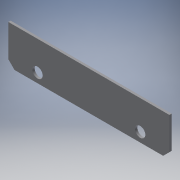
# Autodesk Inventor part: MecanumDriveTrainPlate17-18
Saved by Autodesk Inventor 2017 (Build 210142000, 142)
## iProperties
Created: 2017-09-16
Part Number: MecanumDriveTrainPlate17-18
Material: Generic
Document SubType Name: Modeling
Designer: User
Density: 1 g/cm^3
Appearance: Default
Author: User
Autodesk Inventor part; units mm, degrees
ref_plane "YZ Plane" through (0, 0, 0) normal (1, 0, 0) x (0, 1, 0)
ref_plane "XZ Plane" through (0, 0, 0) normal (0, 1, 0) x (-1, 0, 0)
ref_plane "XY Plane" through (0, 0, 0) normal (0, 0, 1) x (1, 0, 0)
sketch "Sketch1" plane through (0, 0, 0) normal (0, 0, 1) x (1, 0, 0)
  line L0 (0, 0) -> (444.5, 0)
  line L1 (444.5, 0) -> (444.5, 127)
  line L2 (444.5, 127) -> (0, 127)
  line L3 (0, 127) -> (0, 0)
  dimension "d0" = 444.5
  dimension "d1" = 127
  constraints: 8 end point, 2 perpendicular, 1 horizontal, 1 vertical
  measures "d0" distance of L0.start L0.end
  measures "d1" distance of L0.end L1.end
extrude "Extrusion1" add sketch "Sketch1" along normal blind 6.35
sketch "Sketch2" plane through (0, 0, 6.35) normal (0, 0, 1) x (1, 0, 0)
  line L0 (0, 0) -> (444.5, 0) projected
  line L1 (38.0923, 0) -> (0, 38.0919)
  line L2 (0, 127) -> (0, 0) projected
  line L3 (0, 0) -> (444.5, 0) projected
  line L4 (444.5, 0) -> (444.5, 127) projected
  line L5 (444.5, 0) -> (406.4, 0)
  line L6 (444.5, 0) -> (482.6, 0) construction
  line L7 (444.5, 0) -> (444.5, 38.0919)
  line L8 (444.5, 38.0919) -> (406.4086, 0)
  point P0 (419.1126, 0)
  dimension "d19" = 38.1
  dimension "d20" = 180
  constraints: 10 end point, 5 point on line, 3 collinear, 1 horizontal
  measures "d19" distance of L0.end L5.end
  measures "d20" angle of L5 L6
extrude "Extrusion2" cut sketch "Sketch2" against normal blind 50.8
sketch "Sketch3" plane through (0, 0, 6.35) normal (0, 0, 1) x (1, 0, 0)
  line L0 (0, 77.664) -> (80.645, 77.664) construction
  line L1 (444.5, 127) -> (0, 127) projected
  line L2 (80.645, 127) -> (161.29, 127) construction
  circle A0 centre (80.645, 46.355) radius 14.2748
  line L3 (444.5, 38.0919) -> (444.5, 127) projected
  line L4 (444.5, 77.664) -> (525.145, 77.664) construction
  line L5 (444.5, 38.0919) -> (444.5, 127) projected
  line L6 (444.5, 46.355) -> (525.145, 46.355) construction
  circle A1 centre (363.855, 46.355) radius 14.2748
  line L7 (444.5, 127) -> (0, 127) projected
  line L8 (0, 127) -> (0, 38.0919) projected
  circle A2 centre (182.245, 46.355) radius 21.59
  circle A3 centre (262.255, 46.355) radius 21.59
  point P0 (0, 0)
  dimension "d10" = 28.5496
  dimension "d18" = 28.5496
  dimension "d31" = 43.18
  dimension "d32" = 43.18
  constraints: 8 end point, 4 centre point, 4 horizontal, 3 point on line
  measures "d10" diameter of A0
  measures "d18" diameter of A1
  measures "d31" diameter of A2
  measures "d32" diameter of A3
extrude "Extrusion3" cut sketch "Sketch3" against normal blind 50.8 contours A0 | A1
thicken "Thicken1" operation add thickness 20.828 both sides no extend neighbours yes toward (0, 1, 0) faces at (160.8644, 0, 2.1167)
body "Solid1"
